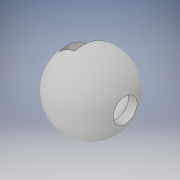
# Autodesk Inventor part: Пирамида
Saved by Autodesk Inventor 2019.3 (Build 233278000, 278)
## iProperties
Created: 2020-04-03
Part Number: Пирамида
Material: Типовые
Document SubType Name: Modeling
Designer: Admin
Density: 1 g/cm^3
Appearance: По умолчанию
Author: Admin
Autodesk Inventor part; units mm, degrees
ref_plane "YZ Plane" through (0, 0, 0) normal (1, 0, 0) x (0, 1, 0)
ref_plane "XZ Plane" through (0, 0, 0) normal (0, 1, 0) x (-1, 0, 0)
ref_plane "XY Plane" through (0, 0, 0) normal (0, 0, 1) x (1, 0, 0)
sketch "Эскиз1" plane through (0, 0, 0) normal (0, 1, 0) x (-1, 0, 0)
  arc A0 (-45, 0) -> (45, 0) centre (0, 0) ccw
  arc A1 (-35, 0) -> (35, 0) centre (0, 0) ccw
  line L0 (45, 0) -> (35, 0)
  line L1 (-35, 0) -> (-45, 0)
  line L2 (63, 0) -> (-63, 0) projected
  dimension "d0" = 45
  dimension "d1" = 35
  constraints: 4 coincident, 4 end point, 4 horizontal alignment, 4 point on circle, 2 centre point, 1 collinear, 1 horizontal
  measures "d0" radius of A0
  measures "d1" radius of A1
revolve "Вращение1" add sketch "Эскиз1" angle 360 about axis through (-10, 0, 0) along (1, 0, 0) contours L1 A1 L0 A0
sketch "Эскиз2" plane through (0, 0, 0) normal (0, 1, 0) x (-1, 0, 0)
  line L0 (30, 10) -> (10, 10)
  line L1 (10, 10) -> (10, -45)
  line L2 (10, -45) -> (30, -45)
  line L3 (30, -45) -> (30, 10)
  line L4 (0, -87.9025) -> (0, 67.1504) projected
  line L5 (63, 0) -> (-63, 0) projected
  circle A0 centre (0, 0) radius 45 projected
  dimension "d3" = 10
  dimension "d4" = 20
  dimension "d5" = 10
  constraints: 8 end point, 2 horizontal, 2 vertical, 1 tangent
  measures "d3" distance between parallel lines of L4 L1
  measures "d4" distance between parallel lines of L3 L1
  measures "d5" distance between parallel lines of L5 L0
extrude "Выдавливание1" cut sketch "Эскиз2" along normal through all both and the other way through all contours L3 L5 L1 L0 | L3 A0 L1 L5 | L3 L2 L1 A0
sketch "Эскиз3" plane through (0, 0, 0) normal (1, 0, 0) x (0, 1, 0)
  circle A0 centre (0, 0) radius 15
  dimension "d8" = 30
  constraints: 1 centre point, 1 coincident
  measures "d8" diameter of A0
extrude "Выдавливание2" cut sketch "Эскиз3" along normal through all
